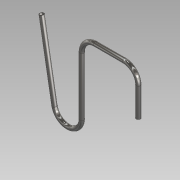
# Autodesk Inventor part: Front support
Saved by Autodesk Inventor 2019 (Build 230136000, 136)
## iProperties
Created: 2020-07-26
Part Number: Front support
Material: Aço inoxidável, polido
Document SubType Name: Modeling
Designer: daniel.regner
Density: 8 g/cm^3
Appearance: Inoxidável - Polido
Author: daniel.regner
Autodesk Inventor part; units mm, degrees
note: some values were not read from the file. Chosen so that the rebuilt part matches the saved one: bend side of "Vergar peça8".
sketch "Esboço10" plane through (0, 0, 0) normal (0, 0, 1) x (1, 0, 0)
  circle A0 centre (0, 0) radius 9.525
  circle A1 centre (0, 0) radius 11.115
  dimension "d35" = 19.05
  dimension "d36" = 1.59
  constraints: 2 centre point, 1 coincident
  measures "d35" diameter of A0
  measures "d36" radial gap between concentric circles of A0 A1
extrude "Extrusão3" add sketch "Esboço10" along normal blind 1350
ref_plane "Plano de trabalho10" through (0, 11.115, 0) normal (0, 1, 0) x (-1, 0, 0)
sketch "Esboço17" plane through (0, 11.115, 0) normal (0, 1, 0) x (-1, 0, 0)
  line L0 (11.115, 0) -> (11.115, 1350) projected
  line L1 (11.115, 150) -> (-11.115, 150)
  line L2 (-11.115, 0) -> (-11.115, 1350) projected
  line L3 (-11.115, 0) -> (11.115, 0) projected
  point P0 (0, 0)
  dimension "d62" = 150
  constraints: 2 end point, 2 point on line, 1 horizontal
  measures "d62" distance between parallel lines of L3 L1
bend part "Vergar peça7" radius 60 angle 90 line through (-11.115, 11.115, 150) along (1, 0, 0) centre toward (0, 1, 0) moving side (0, 0, 1) both sides no
ref_plane "Plano de trabalho11" through (0, -173.1328, 210) normal (0, 0, 1) x (1, 0, 0)
sketch "Esboço18" plane through (0, -173.1328, 210) normal (0, 0, 1) x (1, 0, 0)
  line L0 (11.115, 244.2478) -> (11.115, 1350) projected
  line L1 (11.115, 394.2478) -> (-11.115, 394.2478)
  line L2 (-11.115, 244.2478) -> (-11.115, 1350) projected
  line L3 (11.115, 244.2478) -> (-11.115, 244.2478) projected
  point P0 (0, 173.1328)
  dimension "d65" = 150
  constraints: 2 end point, 2 point on line, 1 horizontal
  measures "d65" distance between parallel lines of L3 L1
bend part "Vergar peça8" radius 60 angle 90 line through (11.115, 221.115, 210) along (-1, 0, 0) centre toward (0, 0, -1) moving side (0, 1, 0) both sides no
ref_plane "Plano de trabalho12" through (0, 303.345, 638.4956) normal (0, 1, 0) x (-1, 0, 0)
sketch "Esboço19" plane through (0, 303.345, 638.4956) normal (0, 1, 0) x (-1, 0, 0)
  line L0 (-11.115, -488.4956) -> (-11.115, -1350) projected
  line L1 (-11.115, -788.4956) -> (11.115, -788.4956)
  line L2 (11.115, -488.4956) -> (11.115, -1350) projected
  line L3 (-11.115, -488.4956) -> (11.115, -488.4956) projected
  point P0 (0, -638.4956)
  dimension "d68" = 300
  constraints: 2 end point, 2 point on line, 1 horizontal
  measures "d68" distance between parallel lines of L1 L3
bend part "Vergar peça9" radius 60 angle 170 line through (11.115, 303.345, -150) along (-1, 0, 0) centre toward (0, 1, 0) moving side (0, 0, -1) both sides no
